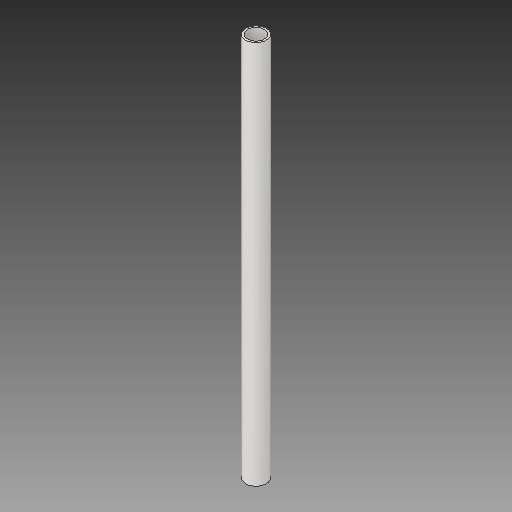
# Autodesk Inventor part: Barrel
Saved by Autodesk Inventor 2017 (Build 210142000, 142)
## iProperties
Created: 2017-10-24
Part Number: Barrel
Material: PVC, Unplasticized
Document SubType Name: Modeling
Designer: Aidan_Moga
Density: 1.29 g/cm^3
Appearance: Smooth - White
Author: Aidan_Moga
Autodesk Inventor part; units mm, degrees
ref_plane "YZ Plane" through (0, 0, 0) normal (1, 0, 0) x (0, 1, 0)
ref_plane "XZ Plane" through (0, 0, 0) normal (0, 1, 0) x (-1, 0, 0)
ref_plane "XY Plane" through (0, 0, 0) normal (0, 0, 1) x (1, 0, 0)
sketch "Sketch1" plane through (0, 0, 0) normal (0, 1, 0) x (-1, 0, 0)
  circle A0 centre (0, 0) radius 20.6375
  circle A1 centre (0, 0) radius 16.8783
  dimension "d0" = 41.275
  dimension "d1" = 33.7566
  constraints: 2 centre point, 2 coincident
  measures "d0" diameter of A0
  measures "d1" diameter of A1
extrude "Extrusion1" add sketch "Sketch1" along normal blind 762
body "Solid1"
